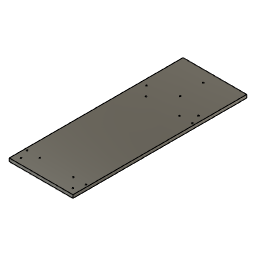
Y Deska v14 (Autodesk Fusion 360 design; units mm, degrees)
Autodesk Fusion 360 part; units mm, degrees
note: some values were not read from the file. Set by a fixed rule: which sketch regions a step uses.
sketch "Sketch1" plane through (0, 0, 0) normal (0, 0, 1) x (1, 0, 0)
  line L0 (0, 0) -> (165, 0)
  line L1 (165, 0) -> (165, 450)
  line L2 (165, 450) -> (0, 450)
  line L3 (0, 450) -> (0, 0)
  circle A0 centre (6, 40) radius 1.75
  circle A1 centre (159, 40) radius 1.75
  circle A2 centre (159, 40) radius 1.75
  circle A3 centre (159, 315) radius 1.75
  circle A4 centre (39, 40) radius 1.75
  circle A5 centre (126, 40) radius 1.75
  circle A6 centre (39, 315) radius 1.75
  circle A7 centre (126, 315) radius 1.75
  circle A8 centre (15, 15) radius 1.75
  circle A9 centre (6, 315) radius 1.75
  circle A10 centre (159, 315) radius 1.75
  circle A11 centre (150, 15) radius 1.75
  circle A12 centre (15, 340) radius 1.75
  circle A13 centre (150, 340) radius 1.75
  circle A14 centre (82.5, 420) radius 1.75
  circle A15 centre (82.5, 360) radius 1.75
  dimension "d1" = 165
  dimension "d2" = 450
  dimension "d5" = 3.5
  dimension "d6" = 6
  dimension "d7" = 40
  dimension "d10" = 153
  dimension "d11" = 275
  dimension "d14" = 153
  dimension "d15" = 275
  dimension "d17" = 3.5
  dimension "d18" = 40
  dimension "d19" = 39
  dimension "d22" = 0
  dimension "d23" = 0
  dimension "d26" = 87
  dimension "d27" = 275
  dimension "d30" = 3.5
  dimension "d31" = 15
  dimension "d32" = 15
  dimension "d33" = 25
  dimension "d36" = 135
  dimension "d37" = 325
  dimension "d40" = 3.5
  dimension "d41" = 82.5
  dimension "d42" = 420
  dimension "d43" = 3.5
  dimension "d44" = 60
  dimension "d45" = 82.5
  constraint horizontal L0
  constraint vertical L1
  constraint horizontal L2
  constraint vertical L3
  constraint coincident L0.start L3.end
  measures "d1" distance of L0.start L0.end
  measures "d2" distance of L0.start L2.end
  measures "d5" diameter of A0
  measures "d6" horizontal distance of L0.start A0.centre
  measures "d7" vertical distance of L0.start A0.centre
  measures "d17" diameter of A4
  measures "d18" vertical distance of L0.start A4.centre
  measures "d19" horizontal distance of L0.start A4.centre
  measures "d30" diameter of A8
  measures "d31" horizontal distance of L0.start A8.centre
  measures "d32" vertical distance of L0.start A8.centre
  measures "d33" vertical distance of A0.centre A8.centre
  measures "d40" diameter of A14
  measures "d41" horizontal distance of L0.start A14.centre
  measures "d42" vertical distance of L0.start A14.centre
  measures "d43" diameter of A15
  measures "d44" distance of A14.centre A15.centre
  measures "d45" horizontal distance of L2.end A15.centre
extrude "Extrude1" add sketch "Sketch1" along normal blind 8 contours L0 L1 L2 L3 | A0 | A1 A2 | A3 A10 | A4 | A5 | A6 | A7 | A8 | A9 | A11 | A12 | A13 | A14 | A15
extrude "Extrude2" cut sketch "Sketch1" along normal blind 30 contours A0 | A1 A2 | A3 A10 | A4 | A5 | A6 | A7
extrude "Extrude3" cut sketch "Sketch1" along normal blind 25 contours A8 | A11 | A12 | A13
extrude "Extrude4" cut sketch "Sketch1" along normal blind 20 contours A14 | A15
